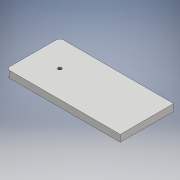
# Autodesk Inventor part: SUPORTE_GUIA_CORREIA_EIXO_Y
Saved by Autodesk Inventor 2018 (Build 220112000, 112)
## iProperties
Created: 2018-10-11
Part Number: SUPORTE_GUIA_CORREIA_EIXO_Y
Material: Genérico
Document SubType Name: Modeling
Designer: Usuario
Density: 1 g/cm^3
Appearance: Padrão
Author: Usuario
Autodesk Inventor part; units mm, degrees
ref_plane "YZ Plane" through (0, 0, 0) normal (1, 0, 0) x (0, 1, 0)
ref_plane "XZ Plane" through (0, 0, 0) normal (0, 1, 0) x (-1, 0, 0)
ref_plane "XY Plane" through (0, 0, 0) normal (0, 0, 1) x (1, 0, 0)
sketch "Esboço1" plane through (0, 0, 0) normal (0, 0, 1) x (1, 0, 0)
  line L0 (-33, -50) -> (-33, 950) projected
  line L1 (47, -50) -> (47, 950) projected
  line L2 (-113, -89.8276) -> (47, -89.8276)
  line L3 (47, -14.8276) -> (-113, -14.8276)
  line L4 (-113, -14.8276) -> (-113, -89.8276)
  line L5 (47, -89.8276) -> (47, -14.8276)
  point P0 (0, 0)
  dimension "d0" = 160
  dimension "d1" = 160
  dimension "d2" = 75
  constraints: 8 end point, 1 collinear, 1 horizontal, 1 parallel, 1 point on line
  measures "d0" distance of L3.start L3.end
  measures "d1" distance of L2.start L2.end
  measures "d2" distance of L3.end L2.start
extrude "Extrusão1" add sketch "Esboço1" along normal blind 9.52
sketch "Esboço11" plane through (0, 0, 9.52) normal (0, 0, 1) x (1, 0, 0)
  circle A0 centre (-75.5, -52.3276) radius 3
  point P0 (0, 0)
  dimension "d95" = 6
  constraints: 1 centre point, 1 coincident
  measures "d95" diameter of A0
hole "Furo2" at (-75.5, -52.3276, 9.52) direction (0, 0, -1) diameter 4.917 end through all thread size "M6x1" class "6H" standard "ANSI Metric M Profile"
fillet "Arredondamento3" radius 5 2 edges at (-113, -89.8276, 4.76) (-113, -14.8276, 4.76)
equation "\"d0\" = d1"
